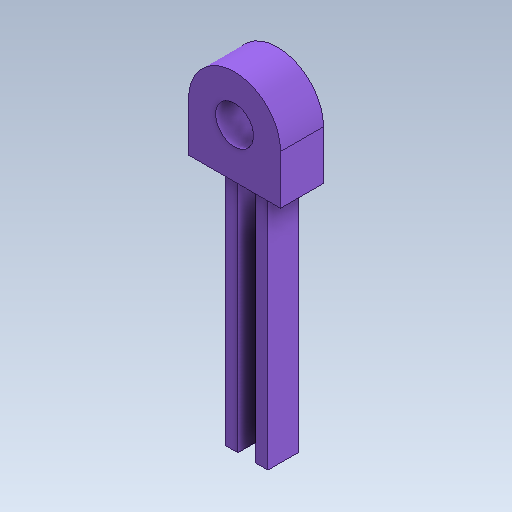
# Autodesk Inventor part: Piston
Saved by Autodesk Inventor 2020 (Build 240168000, 168)
## iProperties
Created: 2020-09-13
Part Number: Piston
Material: Generic
Document SubType Name: Modeling
Designer: Turing
Density: 1 g/cm^3
Appearance: Violet
Mass: 0.260271 g
Surface Area: 4.41653 cm^2
Volume: 0.260271 cm^3
Author: Turing
Autodesk Inventor part; units mm, degrees
ref_plane "YZ Plane" through (0, 0, 0) normal (1, 0, 0) x (0, 1, 0)
ref_plane "XZ Plane" through (0, 0, 0) normal (0, 1, 0) x (-1, 0, 0)
ref_plane "XY Plane" through (0, 0, 0) normal (0, 0, 1) x (1, 0, 0)
sketch "Sketch1" plane through (0, 0, 0) normal (0, 0, 1) x (1, 0, 0)
  line L0 (0, 0) -> (-3.45, 0)
  line L1 (-3.45, 0) -> (-3.45, -20)
  line L2 (-3.45, -20) -> (0, -20)
  line L3 (0, -20) -> (0, 0)
  line L4 (-1.725, -20) -> (-5.425, -20)
  line L5 (-5.425, -20) -> (1.925, -20)
  line L6 (1.925, -20) -> (1.925, -25)
  line L7 (1.925, -25) -> (-5.425, -25)
  line L8 (-5.425, -25) -> (-5.425, -20)
  dimension "d0" = 20
  dimension "d1" = 3.45
  dimension "d2" = 3.7
  dimension "d3" = 7.35
  dimension "d4" = 5
  constraints: 18 end point, 4 parallel, 3 horizontal, 2 perpendicular, 1 midpoint
  measures "d0" distance of L0.end L1.end
  measures "d1" distance of L0.start L0.end
  measures "d2" distance of L4.start L4.end
  measures "d3" distance of L6.end L7.end
  measures "d4" distance of L5.end L6.end
extrude "Extrusion1" add sketch "Sketch1" along normal blind 3.5
sketch "Sketch4" plane through (0, 0, 0) normal (0, 0, -1) x (-1, 0, 0)
  line L0 (0, -20) -> (0, 0) projected
  line L1 (-1.925, -20) -> (0, -20) projected
  line L2 (-1.925, -25) -> (-1.925, -20) projected
  line L3 (5.425, -25) -> (-1.925, -25) projected
  line L4 (5.425, -20) -> (5.425, -25) projected
  line L5 (3.45, -20) -> (5.425, -20) projected
  line L6 (3.45, 0) -> (3.45, -20) projected
  line L7 (0, 0) -> (3.45, 0) projected
  line L8 (3.45, 0) -> (5.475, 0)
  line L9 (0, 0) -> (-2.025, 0)
  line L10 (5.475, 0) -> (-2.025, 0)
  line L11 (-2.025, 0) -> (-2.025, 4)
  line L12 (-2.025, 4) -> (5.475, 4)
  line L13 (5.475, 4) -> (5.475, 0)
  circle A0 centre (1.725, 4) radius 3.75
  circle A1 centre (1.725, 4) radius 1.55
  dimension "d22" = 2.025
  dimension "d23" = 2.025
  dimension "d24" = 7.5
  dimension "d25" = 4
  dimension "d26" = 3.1
  constraints: 12 end point, 3 horizontal, 2 parallel, 1 centre point, 1 coincident, 1 midpoint, 1 perpendicular, 3 other
  measures "d22" distance of L6.start L8.end
  measures "d23" distance of L0.end L9.end
  measures "d24" distance of L11.end L12.end
  measures "d25" distance of L10.end L11.end
  measures "d26" diameter of A1
extrude "Extrusion4" add sketch "Sketch4" against normal up to surface (3.5 mm away) contours L9 L11 A0 L13 L8 L7 | A0 L12 A1 | L12 A1 A0
sketch "Sketch5" plane through (0, 0, 3.5) normal (0, 0, 1) x (1, 0, 0)
  circle A0 centre (-1.725, 4) radius 1.55 projected
  line L0 (0, -20) -> (0, 0) projected
  line L1 (2.025, 0) -> (0, 0) projected
  line L2 (2.025, 4) -> (2.025, 0) projected
  arc A1 (2.025, 4) -> (-5.475, 4) centre (-1.725, 4) ccw projected
  line L3 (-5.475, 0) -> (-5.475, 4) projected
  line L4 (-3.45, 0) -> (-5.475, 0) projected
  line L5 (-3.45, 0) -> (-3.45, -20) projected
  line L6 (-3.45, -20) -> (-5.425, -20) projected
  line L7 (-5.425, -20) -> (-5.425, -25) projected
  line L8 (-5.425, -25) -> (1.925, -25) projected
  line L9 (1.925, -25) -> (1.925, -20) projected
  line L10 (1.925, -20) -> (0, -20) projected
  line L11 (-3.45, -10) -> (0, -10)
  line L12 (-1.725, -10) -> (-1, -10)
  line L13 (-1, -10) -> (-2.45, -10)
  line L14 (-2.45, -10) -> (-2.45, -20)
  line L15 (-2.45, -20) -> (-3.45, -20)
  line L16 (-1, -10) -> (-1, -20)
  line L17 (0, -20) -> (-1, -20)
  dimension "d31" = 1
  dimension "d32" = 1
  constraints: 14 end point, 3 midpoint, 3 perpendicular, 3 point on line
  measures "d31" distance between parallel lines of L14 L5
  measures "d32" distance between parallel lines of L0 L16
extrude "Extrusion5" cut sketch "Sketch5" against normal blind 1.75 contours L10 L9 L8 L7 L6 L15 L14 L11 L16 L17
sketch "Sketch6" plane through (0, 0, 1.75) normal (0, 0, 1) x (1, 0, 0)
  line L0 (1.925, -20) -> (1.925, -25) projected
  line L1 (0, -20) -> (1.925, -20) projected
  line L2 (-1, -20) -> (0, -20) projected
  line L3 (-1, -10) -> (-1, -20) projected
  line L4 (-2.45, -10) -> (-1, -10) projected
  line L5 (-2.45, -20) -> (-2.45, -10) projected
  line L6 (-3.45, -20) -> (-2.45, -20) projected
  line L7 (-5.425, -20) -> (-3.45, -20) projected
  line L8 (-5.425, -25) -> (-5.425, -20) projected
  line L9 (1.925, -25) -> (-5.425, -25) projected
  line L10 (-2.45, -20) -> (-1, -20)
  point P0 (0, 0)
  constraints: 2 end point, 1 horizontal
extrude "Extrusion6" cut sketch "Sketch6" against normal up to surface (1.75 mm away) contours L0 L9 L8 L7 L6 L10 L2 L1
sketch "Sketch7" plane through (-1, -20, 3.5) normal (0, -1, 0) x (1, 0, 0)
  line L0 (1, -3.5) -> (1, 0) projected
  line L1 (0, 0) -> (1, 0) projected
  line L2 (0, 0) -> (0, -1.75) projected
  line L3 (-1.45, -1.75) -> (0, -1.75) projected
  line L4 (-1.45, 0) -> (-1.45, -1.75) projected
  line L5 (-2.45, 0) -> (-1.45, 0) projected
  line L6 (-2.45, -3.5) -> (-2.45, 0) projected
  line L7 (1, -3.5) -> (-2.45, -3.5) projected
  line L8 (-2.45, -3.5) -> (-2.45, 0)
  line L9 (1, 0) -> (-2.45, 0)
  line L10 (-2.45, -3.5) -> (1, -3.5)
  line L11 (1, -3.5) -> (1, 0)
  line L12 (-1.95, -0.5) -> (-1.95, -3)
  line L13 (-1.95, -3) -> (0.5, -3)
  line L14 (0.5, -3) -> (0.5, -0.5)
  line L15 (0.5, -0.5) -> (-1.95, -0.5)
  point P0 (1, -3.5)
  dimension "d37" = 0.5
  constraints: 16 end point, 4 collinear, 3 other
  measures "d37" distance between parallel lines of L9 L15
extrude "Extrusion7" cut sketch "Sketch7" against normal up to surface (20 mm away) contours L7 L6 L5 L4 L15 L12 L13 L14 L2 L1 L0 | L2 L15 L4 L9
sketch "Sketch8" plane through (-2.45, -20, 1.75) normal (0, -1, 0) x (1, 0, 0)
  line L0 (1.95, 1.25) -> (1.45, 1.25) projected
  line L1 (1.45, 1.25) -> (1.45, 0) projected
  line L2 (0, 0) -> (1.45, 0) projected
  line L3 (0, 1.25) -> (0, 0) projected
  line L4 (0, 1.25) -> (-0.5, 1.25) projected
  line L5 (-0.5, 1.25) -> (-0.5, -1.25) projected
  line L6 (-0.5, -1.25) -> (1.95, -1.25) projected
  line L7 (1.95, -1.25) -> (1.95, 1.25) projected
  line L8 (2.45, -1.75) -> (-1, -1.75)
  line L9 (-1, -1.75) -> (-1, 1.75)
  line L10 (-1, 1.75) -> (0.5, 1.75)
  line L11 (0.5, 1.75) -> (0.5, 0.5)
  line L12 (0.5, 0.5) -> (0.95, 0.5)
  line L13 (0.95, 0.5) -> (0.95, 1.75)
  line L14 (0.95, 1.75) -> (2.45, 1.75)
  line L15 (2.45, 1.75) -> (2.45, -1.75)
  line L16 (0, 1.25) -> (0, 1.75)
  line L17 (0, 1.75) -> (-1, 1.75)
  line L18 (-1, 1.75) -> (-1, -1.75)
  line L19 (-1, -1.75) -> (2.45, -1.75)
  line L20 (2.45, -1.75) -> (2.45, 1.75)
  line L21 (2.45, 1.75) -> (1.45, 1.75)
  line L22 (1.45, 0) -> (1.45, 1.75)
  line L23 (0, 0) -> (1.45, 0)
  line L24 (0, 0) -> (0, 1.25)
  point P0 (2.45, -1.75)
  constraints: 34 end point, 4 collinear, 3 perpendicular, 2 point on line, 1 vertical, 7 other
extrude "Extrusion8" add sketch "Sketch8" against normal blind 20 contours L0 L22 L14 L15 L8 L9 L10 L16 L4 L5 L6 L7
sketch "Sketch9" plane through (-2.45, 0, 3) normal (0, 0, 1) x (1, 0, 0)
  line L0 (1.45, -10) -> (1.45, 0) projected
  line L1 (1.45, 0) -> (0, 0) projected
  line L2 (0, 0) -> (0, -10) projected
  line L3 (1.45, -10) -> (0, -10) projected
  line L4 (0, -20) -> (1.45, -20) projected
  line L5 (1.45, -10) -> (1.45, -20) projected
  line L6 (0, -10) -> (1.45, -10) projected
  line L7 (0, -20) -> (0, -10) projected
  point P0 (2.45, 0)
extrude "Extrusion9" cut sketch "Sketch9" against normal up to surface (3 mm away)
sketch "Sketch11" plane through (0, 0, 3.5) normal (0, 0, 1) x (1, 0, 0)
  line L0 (2.025, 0) -> (0, 0) projected
  line L1 (2.025, 4) -> (2.025, 0) projected
  arc A0 (2.025, 4) -> (-5.475, 4) centre (-1.725, 4) ccw projected
  line L2 (-5.475, 0) -> (-5.475, 4) projected
  line L3 (-3.45, 0) -> (-5.475, 0) projected
  line L4 (-3.45, -20) -> (-3.45, 0) projected
  line L5 (-2.45, -20) -> (-3.45, -20) projected
  line L6 (-2.45, -20) -> (-2.45, 0) projected
  line L7 (-1, 0) -> (-2.45, 0) projected
  line L8 (-1, -20) -> (-1, 0) projected
  line L9 (0, -20) -> (-1, -20) projected
  line L10 (0, -20) -> (0, 0) projected
  circle A1 centre (-1.725, 4) radius 1.55 projected
  line L11 (-1, 0) -> (0, 0)
  line L12 (-2.45, 0) -> (-3.45, 0)
  point P0 (0, 0)
  constraints: 4 end point, 2 collinear
extrude "Extrusion11" cut sketch "Sketch11" against normal blind 1 contours L10 L9 L8 L11 | L6 L5 L4 L12
equation "\"d23\" = d22"
equation "\"d32\" = d31"
body "Solid1"
